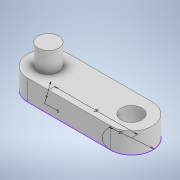
# Autodesk Inventor part: Part1
Saved by Autodesk Inventor 2022 (Build 260153000, 153)
## iProperties
Created: 2022-03-13
Part Number: Part1
Material: Generic
Document SubType Name: Modeling
Designer: br4ch
Density: 1 g/cm^3
Appearance: Default
Author: br4ch
Autodesk Inventor part; units mm, degrees
ref_plane "YZ Plane" through (0, 0, 0) normal (1, 0, 0) x (0, 1, 0)
ref_plane "XZ Plane" through (0, 0, 0) normal (0, 1, 0) x (-1, 0, 0)
ref_plane "XY Plane" through (0, 0, 0) normal (0, 0, 1) x (1, 0, 0)
sketch "Sketch1" plane through (0, 0, 0) normal (0, 1, 0) x (-1, 0, 0)
  line L0 (-2, -2) -> (-22, -2) construction
  line L1 (-2, 3) -> (-22, 3)
  line L2 (-22, -7) -> (-2, -7)
  arc A0 (-2, -7) -> (-2, 3) centre (-2, -2) ccw
  arc A1 (-22, 3) -> (-22, -7) centre (-22, -2) ccw
  circle A2 centre (-2, -2) radius 2.5
  circle A3 centre (-22, -2) radius 2.5
  point P0 (0, 0)
  point P1 (-12, -2)
  dimension "d0" = 20
  dimension "d1" = 10
  dimension "d2" = 5
  constraints: 8 end point, 4 centre point, 4 point on circle, 4 tangent, 2 coincident, 1 equal radius, 1 horizontal, 1 midpoint, 1 parallel
  measures "d0" distance of L0.start L0.end
  measures "d1" diameter of A1
  measures "d2" diameter of A2
extrude "Extrusion1" add sketch "Sketch1" along normal blind 5 contours A0 L2 A1 L1 | A2
sketch "Sketch2" plane through (0, 5, 0) normal (0, 1, 0) x (1, 0, 0)
  circle A0 centre (2, 2) radius 2.5 projected
  point P0 (0, 0)
extrude "Extrusion3" add sketch "Sketch2" along normal blind 5
body "Solid1"
